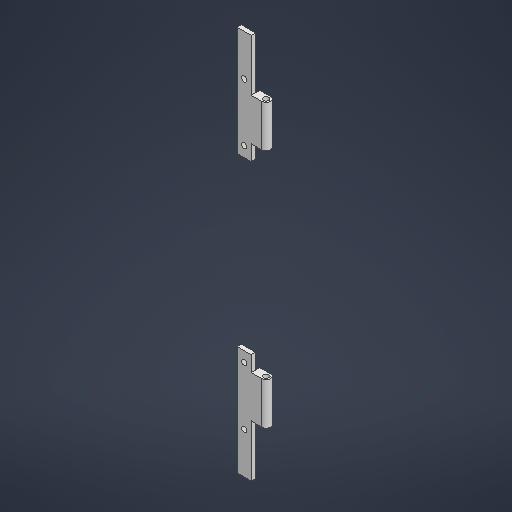
# Autodesk Inventor part: mocowaniedoplugu
Saved by Autodesk Inventor 2026.2 (Build 302298010, 298A)
## iProperties
Created: 2026-09-28
Part Number: mocowaniedoplugu
Material: Generic
Document SubType Name: Modeling
Designer: karol
Density: 1 g/cm^3
Appearance: Default
Author: karol
Autodesk Inventor part; units mm, degrees
ref_plane "YZ Plane" through (0, 0, 0) normal (1, 0, 0) x (0, 1, 0)
ref_plane "XZ Plane" through (0, 0, 0) normal (0, 1, 0) x (-1, 0, 0)
ref_plane "XY Plane" through (0, 0, 0) normal (0, 0, 1) x (1, 0, 0)
sketch "Sketch1" plane through (0, 0, 0) normal (0, 0, 1) x (1, 0, 0)
  circle A0 centre (3.25, 19.2) radius 1.25 projected
  circle A1 centre (3.25, 46.2) radius 1.25 projected
  circle A2 centre (3.25, 133.8) radius 1.25 projected
  circle A3 centre (3.25, 160.8) radius 1.25 projected
  line L0 (0, 0) -> (6.5, 0) projected
  line L1 (6.5, 0) -> (6.5, 180) projected
  line L2 (0, 180) -> (6.5, 180) projected
  line L3 (0, 0) -> (0, 180) projected
  line L4 (6.5, 180) -> (0, 180)
  line L5 (0, 180) -> (0, 129)
  line L6 (0, 129) -> (6.5, 129)
  line L7 (6.5, 129) -> (6.5, 180)
  line L8 (6.5, 0) -> (0, 0)
  line L9 (0, 0) -> (0, 51)
  line L10 (0, 51) -> (6.5, 51)
  line L11 (6.5, 51) -> (6.5, 0)
  line L12 (6.5, 155.8) -> (13.5, 155.8)
  line L13 (13.5, 155.8) -> (13.5, 136.2)
  line L14 (13.5, 136.2) -> (6.5, 136.2)
  line L15 (6.5, 136.2) -> (6.5, 155.8)
  line L16 (6.5, 43.8) -> (13.5, 43.8)
  line L17 (13.5, 43.8) -> (13.5, 24.2)
  line L18 (13.5, 24.2) -> (6.5, 24.2)
  line L19 (6.5, 24.2) -> (6.5, 43.8)
  dimension "d0" = 51
  dimension "d1" = 51
  dimension "d2" = 7
  dimension "d3" = 19.6
  dimension "d4" = 24.2
  dimension "d5" = 7
  dimension "d6" = 19.6
  dimension "d7" = 24.2
  constraints: 32 end point, 8 parallel, 4 horizontal, 4 perpendicular, 4 point on line
  measures "d0" distance of L5.end L4.end
  measures "d1" distance of L8.end L9.end
  measures "d2" distance of L13.end L14.end
  measures "d3" distance of L12.end L13.end
  measures "d4" distance between parallel lines of L2 L12
  measures "d5" distance of L17.end L18.end
  measures "d6" distance of L16.end L17.end
  measures "d7" distance between parallel lines of L18 L0
extrude "Extrusion1" add sketch "Sketch1" along normal blind 2 contours L3 L10 L1 L0 | L1 L16 L17 L18 | L3 L2 L1 L6 | L1 L12 L13 L14
sketch "Sketch2" plane through (0, 0, 0) normal (0, 0, -1) x (-1, 0, 0)
  line L0 (0, 51) -> (0, 0) projected
  line L1 (-6.5, 51) -> (0, 51) projected
  line L2 (-6.5, 43.8) -> (-6.5, 51) projected
  line L3 (-13.5, 43.8) -> (-6.5, 43.8) projected
  line L4 (-13.5, 24.2) -> (-13.5, 43.8) projected
  line L5 (-6.5, 24.2) -> (-13.5, 24.2) projected
  line L6 (-6.5, 0) -> (-6.5, 24.2) projected
  line L7 (0, 0) -> (-6.5, 0) projected
  circle A0 centre (-3.25, 19.2) radius 1.25 projected
  circle A1 centre (-3.25, 46.2) radius 1.25 projected
  line L8 (-6.5, 129) -> (-6.5, 136.2) projected
  line L9 (0, 129) -> (-6.5, 129) projected
  line L10 (0, 180) -> (0, 129) projected
  line L11 (-6.5, 180) -> (0, 180) projected
  line L12 (-6.5, 155.8) -> (-6.5, 180) projected
  line L13 (-13.5, 155.8) -> (-6.5, 155.8) projected
  line L14 (-13.5, 136.2) -> (-13.5, 155.8) projected
  line L15 (-6.5, 136.2) -> (-13.5, 136.2) projected
  circle A2 centre (-3.25, 133.8) radius 1.25 projected
  circle A3 centre (-3.25, 160.8) radius 1.25 projected
  line L16 (-6.5, 136.2) -> (-6.5, 155.8)
  line L17 (-6.5, 24.2) -> (-6.5, 43.8)
  constraints: 4 end point, 1 collinear, 1 perpendicular
extrude "Extrusion2" add sketch "Sketch2" along normal blind 2 contours L17 L5 L4 L3 | L15 L14 L13 L16
fillet "Fillet1" radius 2 4 edges at (13.5, 34, -2) (13.5, 34, 2) (13.5, 146, -2) (13.5, 146, 2)
sketch "Sketch3" plane through (6.5, 155.8, 0) normal (0, 1, 0) x (1, 0, 0)
  circle A0 centre (5, 0) radius 1.3
  arc A1 (5, -2) -> (5, 2) centre (5, 0) ccw projected
  point P0 (-6.5, 0)
  dimension "d13" = 2.6
  constraints: 1 centre point, 1 concentric
  measures "d13" diameter of A0
extrude "Extrusion3" cut sketch "Sketch3" against normal blind 20
sketch "Sketch4" plane through (6.5, 43.8, 0) normal (0, 1, 0) x (1, 0, 0)
  circle A0 centre (5, 0) radius 1.3 projected
  point P0 (-6.5, 0)
extrude "Extrusion4" cut sketch "Sketch4" against normal blind 20
body "Solid1"
